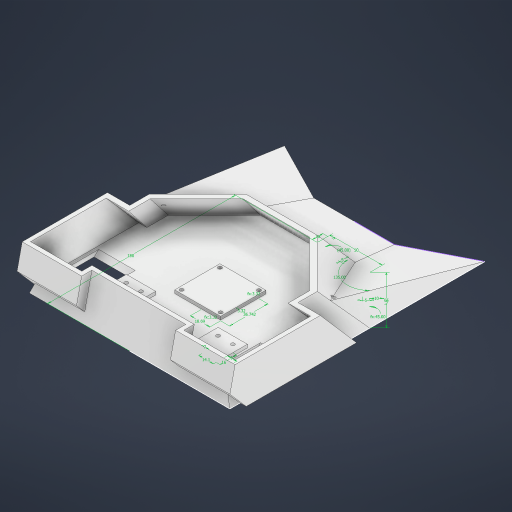
# Autodesk Inventor part: chassis
Saved by Autodesk Inventor 2023 (Build 270158000, 158)
## iProperties
Created: 2022-06-22
Part Number: chassis
Material: ABS Plastic
Document SubType Name: Modeling
Designer: Dan
Density: 1.06 g/cm^3
Appearance: Smooth - White
Author: Dan
Autodesk Inventor part; units mm, degrees
ref_plane "YZ Plane" through (0, 0, 0) normal (1, 0, 0) x (0, 1, 0)
ref_plane "XY Plane" through (0, 0, 0) normal (0, 0, 1) x (1, 0, 0)
sketch "Base Sketch" plane through (0, 0, 0) normal (0, 1, 0) x (-1, 0, 0)
  line L0 (0, -90) -> (0, 90)
  line L1 (0, -90) -> (-50, -90)
  line L2 (-50, -90) -> (-95.961941, -44.038059)
  line L3 (-95.961941, -44.038059) -> (-95.961941, 90)
  line L4 (-95.961941, 90) -> (0, 90)
  point P0 (0, 0)
  dimension "d0" = 180
  dimension "d1" = 50
  dimension "d2" = 65
  dimension "d3" = 135
  constraints: 10 end point, 2 midpoint, 2 perpendicular, 1 horizontal, 1 vertical
  measures "d0" distance of L0.start L0.end
  measures "d1" distance of L0.start L1.end
  measures "d2" distance of L1.end L2.end
  measures "d3" angle of L1 L2
ref_plane "Top Plane" through (0, 40, 0) normal (0, 1, 0) x (-1, 0, 0)
sketch "Sketch3" plane through (0, 40, 0) normal (0, 1, 0) x (-1, 0, 0)
  line L0 (0, -90) -> (0, 90)
  line L1 (0, -90) -> (-50, -90)
  line L2 (-50, -90) -> (-95.961941, -44.038059)
  line L3 (-95.961941, -44.038059) -> (-95.961941, 90)
  line L4 (-95.961941, 90) -> (0, 90)
  line L5 (-34.065753, -55.907511) -> (0, -55.907511)
  line L6 (0, 81.084403) -> (-80.650201, 81.084403)
  line L7 (-80.650201, 81.084403) -> (-80.650201, -9.323063)
  line L8 (-80.650201, -9.323063) -> (-34.065753, -55.907511)
  point P0 (0, 0)
  constraints: 8 end point, 4 parallel, 2 point on line, 1 horizontal, 1 vertical
loft "Body Loft" add profiles "Base Sketch", "Sketch3" contours all / L5 L8 L7 L6 L0
ref_plane "Wheel-Plane" through (60, 0, -90) normal (-1, 0, 0) x (0, 0, 1)
sketch "Sketch4" plane through (60, 0, -90) normal (-1, 0, 0) x (0, 0, 1)
  line L0 (45.961941, 0) -> (180, 0)
  line L1 (140, -7) -> (140, 63) construction
  circle A0 centre (140, 28) radius 35
  point P0 (90, 0)
  dimension "wheeld" = 70
  dimension "rideh" = 7
  dimension "d14" = 70
  dimension "d17" = 40
  constraints: 2 end point, 1 centre point, 1 midpoint, 1 vertical
  measures "wheeld" distance of L1.start L1.end
  measures "rideh" distance from line of L1.start L0
  measures "d14" diameter of A0
  measures "d17" distance from line of L0.end L1
extrude "Wheel Extrusion" add sketch "Sketch4" against normal blind 35 separate body
sketch "Sketch5" plane through (95, 28, 50) normal (1, 0, 0) x (0, 0, -1)
  circle A0 centre (0, 0) radius 35 construction
  line L0 (-40.851964, 12) -> (40.851964, 12)
  line L1 (40.851964, 12) -> (75.566959, -28)
  line L2 (-40, -28) -> (94.038059, -28)
  line L3 (94.038059, -28) -> (59.323063, 12) construction
  circle A1 centre (0, 0) radius 35
  line L4 (0, 35) -> (0, 40.033944) construction
  line L5 (-45.769406, -10.062202) -> (-30.201641, -28)
  line L6 (-40.851964, 12) -> (-45.769406, -10.062202)
  line L7 (75.566959, -28) -> (-30.201641, -28)
  line L8 (-31.084403, 12) -> (59.323063, 12)
  line L9 (-40, -28) -> (-31.084403, 12) construction
  point P0 (50, -28)
  point P1 (0, 12)
  point P2 (-21.084403, 9.5)
  point P3 (-37.997776, -19.016983)
  point P4 (-21.084403, 9.5)
  dimension "d18" = 130.954
  constraints: 12 end point, 4 point on line, 2 parallel, 1 collinear, 1 horizontal, 1 midpoint, 1 vertical, 1 vertical alignment, 5 other
  measures "d18" angle of L0 L1
extrude "Wheelwell Extrusion" add sketch "Sketch5" along normal blind 7 and the other way blind 50 separate body contours L0 A1 L2 L5 L6 | L0 A1 L2 | L0 L1 L2 A1
combine bodies "Body Combine" operation type add bodies to combine 3 1
sketch "Ramp Base Sketch" plane through (0, 0, 0) normal (0, 1, 0) x (-1, 0, 0)
  line L0 (0, -125.203772) -> (-38.662053, -125.203772)
  line L1 (-38.662053, -125.203772) -> (-95.961941, -154.496231)
  line L2 (-95.961941, -154.496231) -> (-95.961941, -44.038059)
  line L3 (-50, -90) -> (0, -90)
  line L4 (-95.961941, -44.038059) -> (-50, -90)
  line L5 (-95.961941, 90) -> (-95.961941, -44.038059)
  line L6 (0, -90) -> (0, -55.907511)
  line L7 (0, -90) -> (0, -125.203772)
  point P0 (0, 0)
  constraints: 8 end point, 2 vertical, 1 horizontal
sketch "Inner Ramp CS" plane through (0, 0, -90) normal (-1, 0, 0) x (0, 0, 1)
  line L0 (-35.203772, 0) -> (12.745324, 11.870586)
  line L1 (0, 0) -> (34.092489, 40) construction
  line L2 (0, 0) -> (-35.203772, 0)
  line L3 (1.52214, -1.297339) -> (35.614629, 38.702661)
  line L4 (45.961941, 0) -> (0, 0)
  line L5 (2.627878, 0) -> (-35.203772, 0)
  point P0 (90, 0)
  point P1 (9.414663, 11.046027)
  dimension "d107" = 2
  constraints: 6 end point, 5 point on line, 1 collinear, 1 parallel
  measures "d107" distance between parallel lines of L1 L3
ref_plane "Mid Ramp Plane" through (0, 0, -125.203772) normal (0, -0.9706958, 0.2403117) x (1, 0, 0)
sketch "Mid Ramp Construction" plane through (0, 0, -125.203772) normal (0, -0.9706958, 0.2403117) x (1, 0, 0)
  line L0 (0, 166.450502) -> (102, 166.450502)
  line L1 (86.165237, 106.497774) -> (45.599747, 45.965416) construction
  line L2 (45.599747, 45.965416) -> (0, 45.965416)
  line L3 (0, 45.965416) -> (0, 166.450502)
  line L4 (83.935775, 130.733759) -> (86.165237, 106.497774) construction
  line L5 (102, 130.733759) -> (83.935775, 130.733759)
  line L6 (102, 166.450502) -> (102, 130.733759)
  line L7 (95, 145.139589) -> (60, 145.139589)
  line L8 (60, 145.139589) -> (60, 208.456989)
  line L9 (60, 208.456989) -> (95, 208.456989)
  line L10 (95, 208.456989) -> (95, 145.139589)
  point P0 (0, 121.534773)
  point P1 (80.650201, 166.450502)
ref_plane "Outer Ramp Plane" through (95.961941, 0, -154.496231) normal (-0.1135345, 0.9683939, -0.2220884) x (-0.8903978, 0, 0.4551831)
sketch "Outer Ramp Construction" plane through (95.961941, 0, -154.496231) normal (-0.1135345, 0.9683939, -0.2220884) x (-0.8903978, 0, 0.4551831)
  line L0 (72.609886, 160.368193) -> (187.165419, 160.368193)
  line L1 (187.165419, 160.368193) -> (116.50932, 17.644663) construction
  line L2 (116.50932, 17.644663) -> (78.48538, 44.285783) construction
  line L3 (78.48538, 44.285783) -> (72.31756, 120.071559)
  line L4 (72.31756, 120.071559) -> (84.410688, 140.150234)
  line L5 (84.410688, 140.150234) -> (68.242585, 151.546357)
  line L6 (68.242585, 151.546357) -> (72.609886, 160.368193)
  ellipse E0 centre (236.611027, 112.257735) end of major axis (512.885958, -24.513748) minor radius 35 (78.842887, 157.078356) -> (109.476635, 139.556039) ccw
  line L7 (78.842887, 157.078356) -> (105.310479, 210.542221)
  ellipse E1 centre (236.611027, 112.257735) end of major axis (512.885958, -24.513748) minor radius 35 (137.818483, 196.805853) -> (105.310479, 210.542221) ccw
  line L8 (137.818483, 196.805853) -> (109.476635, 139.556039)
  point P0 (155.768382, 90.91558)
  point P1 (96.587706, 160.368193)
  constraints: 2 other
ref_plane "Side Ramp Plane" through (95.961941, 0, 90) normal (0.9339145, 0.3574964, 0) x (0, 0, -1)
sketch "Side Ramp CS" plane through (95.961941, 0, 90) normal (0.9339145, 0.3574964, 0) x (0, 0, -1)
  line L0 (108.046099, 32.068214) -> (244.496231, 0)
  line L1 (134.038059, 0) -> (99.323063, 42.830472) construction
  line L2 (244.496231, 0) -> (134.038059, 0)
  line L3 (131.463612, 0) -> (104.865858, 32.815628)
  line L4 (108.046099, 32.068214) -> (104.865858, 32.815628)
  line L5 (134.038059, 0) -> (131.463612, 0)
  point P0 (90, 34.306048)
  dimension "d110" = 2
  constraints: 8 end point, 2 collinear, 1 parallel
  measures "d110" distance between parallel lines of L1 L3
ref_plane "Mid Ramp CS Plane" through (38.662053, 0, -125.203772) normal (0.8015499, 0.5393286, -0.2581521) x (0.1492426, 0.2376203, 0.9598246)
sketch "Sketch20" plane through (38.662053, 0, -125.203772) normal (0.8015499, 0.5393286, -0.2581521) x (0.1492426, 0.2376203, 0.9598246)
  line L0 (46.486031, 0) -> (0, 0)
  line L1 (0, 0) -> (35.48155, 10.436197)
  line L2 (35.48155, 10.436197) -> (46.486031, 0) construction
  line L3 (49.392487, 0) -> (37.699971, 11.088702)
  line L4 (35.48155, 10.436197) -> (37.699971, 11.088702)
  line L5 (46.486031, 0) -> (49.392487, 0)
  point P0 (114.403635, -8.616313)
  dimension "d109" = 2
  constraints: 12 end point, 2 collinear, 1 horizontal, 1 parallel
  measures "d109" distance between parallel lines of L2 L3
loft "Ramp Loft Mid" add profiles "Inner Ramp CS", "Sketch20" separate body
loft "Ramp Loft outer" add profiles "Side Ramp CS" bodies 4 section 1 edges at (44.331027, 0, -107.601886) (50.354442, 0, -88.899474) (45.816631, 11.391343, -79.190493) (42.1309, 5.523013, -102.894554) (48.371199, 5.86833, -82.797298)
shell "Body Shell" thickness 4 removed faces 2 at (0, 3.333333, 15.75037) at (26.8834, 40, 11.441643) bodies 3
ref_plane "Motor Mount Plane" through (49, 4, 66.14331) normal (0, 1, 0) x (-1, 0, 0)
combine bodies "Wheel Hole" operation type subtract main body 3 bodies to subtract 2 keep tools yes
sketch "Mount Holes" plane through (49, 0, 66.14331) normal (0, 1, 0) x (-1, 0, 0)
  line L0 (12.1, -8.14331) -> (12.1, -24.14331) construction
  line L1 (-2, -8.14331) -> (12.1, -8.14331) construction
  line L2 (-2, -24.14331) -> (12.1, -24.14331) construction
  line L3 (-2, -24.14331) -> (-2, -8.14331) construction
  line L4 (-11, -16.14331) -> (-2, -16.14331) construction
  line L5 (19.1, -1.14331) -> (19.1, -31.14331)
  line L6 (19.1, -31.14331) -> (-9, -31.14331)
  line L7 (-9, -31.14331) -> (-9, -1.14331)
  line L8 (-9, -1.14331) -> (19.1, -1.14331)
  line L9 (49, 18.866975) -> (49, -147.478305)
  line L10 (49, -41.414358) -> (26.99, -41.414358)
  line L11 (26.99, -41.414358) -> (26.99, -84.796358)
  line L12 (26.99, -84.796358) -> (49, -84.796358)
  line L13 (49, -84.796358) -> (49, -41.414358)
  line L14 (30.31, -81.476358) -> (30.31, -44.734358) construction
  line L15 (30.31, -44.734358) -> (49, -44.734358) construction
  line L16 (49, -81.476358) -> (30.31, -81.476358) construction
  point P0 (49, -66.14331)
  point P1 (49, -84.796358)
  point P2 (37.995, -41.414358)
  dimension "d87" = 14.1
  dimension "d88" = 16
  dimension "d139" = 9
  dimension "d140" = 7
  dimension "d145" = 3.32
  dimension "d146" = 36.742
  dimension "d147" = 3.32
  dimension "d148" = 3.32
  dimension "d149" = 18.69
  constraints: 32 end point, 3 horizontal, 3 parallel, 3 perpendicular, 3 point on line, 2 coincident, 2 midpoint, 2 vertical, 3 other
  measures "d87" distance of L1.start L0.start
  measures "d88" distance of L2.start L1.start
  measures "d139" distance of L4.start L4.end
  measures "d140" distance between parallel lines of L5 L0
  measures "d145" distance between parallel lines of L11 L14
  measures "d146" distance of L14.start L14.end
  measures "d147" distance from line of point (37.995, -41.414) L15
  measures "d148" distance between parallel lines of L12 L16
  measures "d149" distance of L14.end L15.end
extrude "Motor Mount" add sketch "Mount Holes" along normal blind 7 bodies 3
hole "Motor Holes" at (36.9, 0, 58) at (36.9, 0, 42) at (51, 0, 58) at (51, 0, 42) at (18.69, 0, 21.408952) at (18.69, 0, -15.333048) direction (0, 1, 0) diameter 3.4 depth 7 counterbore diameter 6.5 counterbore depth 3.4 bodies 3 clearance for "Socket Head Cap Screw ISO 4762" size "M3" standard "ISO"
sketch "Ramp Tab Sketch" plane through (0, 0, -90) normal (0, -1, 0) x (1, 0, 0)
  line L0 (0, -10) -> (5, -10)
  line L1 (5, -10) -> (20, 5)
  line L2 (50, 0) -> (0, 0) construction
  line L3 (95.961941, 45.961941) -> (50, 0)
  line L4 (0, 0) -> (0, 34.092489)
  line L5 (0, 0) -> (0, -10)
  line L6 (83.417916, 40.488984) -> (83.417916, 19.275781)
  line L7 (83.417916, 19.275781) -> (79.882382, 15.740247)
  line L8 (79.882382, 15.740247) -> (72.811315, 22.811315) construction
  line L9 (55.133645, 12.204713) -> (76.346848, 12.204713)
  line L10 (76.346848, 12.204713) -> (79.882382, 15.740247)
  line L11 (48.422197, 5) -> (0, 5)
  line L12 (3, 5) -> (3, 36.092489)
  line L13 (94.643858, 51.714926) -> (47.562584, 4.633652)
  point P0 (0, 90)
  point P1 (48.422197, 0)
  point P2 (94.524512, 44.524512)
  point P3 (51.098118, 1.098118)
  point P4 (83.417916, 33.417916)
  point P5 (62.204713, 12.204713)
  point P6 (62.204713, 12.204713)
  dimension "d75" = 5
  dimension "d76" = 10
  dimension "d77" = 45
  dimension "d78" = 45
  dimension "d80" = 5
  dimension "d81" = 10
  dimension "d82" = 5
  dimension "d83" = 5
  constraints: 22 end point, 9 point on line, 3 parallel, 2 symmetric about line, 1 horizontal, 1 perpendicular, 1 vertical
  measures "d75" distance of L0.start L0.end
  measures "d76" distance of L2.end L0.start
  measures "d77" angle of L2 L1
  measures "d78" angle of L3 L6
  measures "d80" distance of L6.end L7.end
  measures "d81" distance of L7.end L8.end
  measures "d82" distance between parallel lines of L2 L11
  measures "d83" distance between parallel lines of L3 L13
extrude "Ramp Tab" add sketch "Ramp Tab Sketch" against normal up to surface (4 mm away) bodies 3
ref_plane "Work Plane10" through (79.212772, 40, -10.760493) normal (0.5296887, 0.6624649, -0.5296887) x (0.4684334, -0.7490929, -0.4684334)
sketch "Sketch21" plane through (79.212772, 40, -10.760493) normal (0.5296887, 0.6624649, -0.5296887) x (0.4684334, -0.7490929, -0.4684334)
  point P0 (-12.182767, 48.403071)
  point P1 (15.679941, 7.852119)
hole "Hole2" at (81.005494, 28.254267, -23.657787) direction (-0.5296887, -0.6624649, 0.5296887) diameter 3.4 depth 4 bodies 3 clearance for "Flat Head Machine Screw" size "M3" standard "Ansi Metric M Profile"
hole "Hole3" at (81.005494, 28.254267, -23.657787) direction (0.5296887, 0.6624649, -0.5296887) diameter 3.4 depth 14.75 bodies 4 clearance for "Flat Head Machine Screw" size "M3" standard "Ansi Metric M Profile"
combine bodies "Final Ramp Fitting (Work above this)" operation type subtract main body 4 bodies to subtract 3 keep tools yes
mirror "Mirror2" about plane through (0, 0, 0) normal (1, 0, 0) bodies 3 4
equation "\"d14\" = wheeld"
